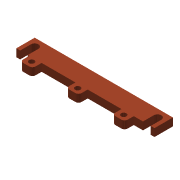
# Autodesk Inventor part: RodHolderV4
Saved by Autodesk Inventor 2013 (Build 170138000, 138)
## iProperties
Created: 2013-04-30
Part Number: RodHolderV4
Material: Copper
Document SubType Name: Modeling
Designer: 120pa
Density: 1 g/cm^3
Author: 120pa
Autodesk Inventor part; units mm, degrees
ref_plane "YZ Plane" through (0, 0, 0) normal (1, 0, 0) x (0, 1, 0)
ref_plane "XZ Plane" through (0, 0, 0) normal (0, 1, 0) x (-1, 0, 0)
ref_plane "XY Plane" through (0, 0, 0) normal (0, 0, 1) x (1, 0, 0)
sketch "Sketch1" plane through (0, 0, 0) normal (0, 1, 0) x (-1, 0, 0)
  line L0 (26.0651, -39.5603) -> (116.0651, -39.5603)
  line L1 (116.0651, -39.5603) -> (116.0651, -27.5603)
  line L2 (116.0651, -27.5603) -> (26.0651, -27.5603)
  line L3 (26.0651, -27.5603) -> (26.0651, -39.5603)
  line L4 (39.5651, -27.5603) -> (47.5651, -27.5603)
  line L5 (47.5651, -27.5603) -> (47.5651, -21.5603)
  line L6 (47.5651, -21.5603) -> (39.5651, -21.5603)
  line L7 (39.5651, -21.5603) -> (39.5651, -27.5603)
  line L8 (69.5651, -27.5603) -> (77.5651, -27.5603)
  line L9 (77.5651, -27.5603) -> (77.5651, -21.5603)
  line L10 (77.5651, -21.5603) -> (69.5651, -21.5603)
  line L11 (69.5651, -21.5603) -> (69.5651, -27.5603)
  line L12 (99.5651, -27.5603) -> (107.5651, -27.5603)
  line L13 (107.5651, -27.5603) -> (107.5651, -21.5603)
  line L14 (107.5651, -21.5603) -> (99.5651, -21.5603)
  line L15 (99.5651, -21.5603) -> (99.5651, -27.5603)
  point P0 (0, 0)
  dimension "d0" = 90
  dimension "d3" = 12
  dimension "d4" = 21.5
  dimension "d5" = 30
  dimension "d6" = 30
  dimension "d7" = 6
  dimension "d8" = 6
  dimension "d9" = 6
  dimension "d10" = 8
  dimension "d11" = 8
  dimension "d12" = 8
  constraints: 32 end point, 8 parallel, 4 horizontal, 4 perpendicular, 3 point on line
  measures "d0" distance of L0.start L0.end
  measures "d3" distance of L0.end L1.end
  measures "d4" distance between parallel lines of L3 L5
  measures "d5" distance between parallel lines of L5 L9
  measures "d6" distance between parallel lines of L9 L13
  measures "d7" distance of L6.end L4.start
  measures "d8" distance of L10.end L8.start
  measures "d9" distance of L14.end L12.start
  measures "d10" distance of L5.end L6.end
  measures "d11" distance of L9.end L10.end
  measures "d12" distance of L13.end L14.end
extrude "Extrusion1" add sketch "Sketch1" along normal blind 5
fillet "Fillet1" radius 2 1 edges at (-99.5651, 2.5, -21.5603)
fillet "Fillet2" radius 2 1 edges at (-107.5651, 2.5, -21.5603)
fillet "Fillet3" radius 2 1 edges at (-77.5651, 2.5, -21.5603)
fillet "Fillet4" radius 2 1 edges at (-69.5651, 2.5, -21.5603)
fillet "Fillet5" radius 2 1 edges at (-47.5651, 2.5, -21.5603)
fillet "Fillet6" radius 2 1 edges at (-39.5651, 2.5, -21.5603)
sketch "Sketch2" plane through (0, 0, 0) normal (0, -1, 0) x (1, 0, 0)
  line L0 (-39.5651, -23.5603) -> (-39.5651, -27.5603) projected
  circle A0 centre (-103.5651, -25.0603) radius 1.75
  circle A1 centre (-73.5651, -25.0603) radius 1.75
  circle A2 centre (-43.5651, -25.0603) radius 1.75
  line L1 (-69.5651, -27.5603) -> (-47.5651, -27.5603) projected
  line L2 (-69.5651, -23.5603) -> (-69.5651, -27.5603) projected
  line L3 (-99.5651, -27.5603) -> (-77.5651, -27.5603) projected
  line L4 (-99.5651, -23.5603) -> (-99.5651, -27.5603) projected
  line L5 (-39.5651, -27.5603) -> (-26.0651, -27.5603) projected
  point P0 (0, 0)
  dimension "d23" = 3.5
  dimension "d29" = 3.5
  dimension "d30" = 3.5
  dimension "d47" = 2.5
  dimension "d48" = 4
  dimension "d49" = 2.5
  dimension "d50" = 4
  dimension "d51" = 2.5
  dimension "d52" = 4
  constraints: 3 centre point
  measures "d23" diameter of A0
  measures "d29" diameter of A1
  measures "d30" diameter of A2
  measures "d47" distance from line of L3 A0.centre
  measures "d48" distance from line of L4 A0.centre
  measures "d49" distance from line of L1 A1.centre
  measures "d50" distance from line of A1.centre L2
  measures "d51" distance from line of L5 A2.centre
  measures "d52" distance from line of L0 A2.centre
extrude "Extrusion2" cut sketch "Sketch2" against normal blind 10
sketch "Sketch4" plane through (0, 5, 0) normal (0, 1, 0) x (1, 0, 0)
  line L0 (-26.0651, 27.5603) -> (-26.0651, 39.5603) projected
  line L1 (-26.0651, 39.5603) -> (-116.0651, 39.5603) projected
  line L2 (-116.0651, 39.5603) -> (-116.0651, 27.5603) projected
  arc A0 (-108.5651, 34.5603) -> (-113.5651, 34.5603) centre (-111.0651, 34.5603) ccw
  arc A1 (-28.5651, 34.5603) -> (-33.5651, 34.5603) centre (-31.0651, 34.5603) ccw
  line L3 (-113.5651, 27.5603) -> (-108.5651, 27.5603)
  line L4 (-108.5651, 27.5603) -> (-108.5651, 34.5603)
  line L5 (-113.5651, 34.5603) -> (-113.5651, 27.5603)
  line L6 (-33.5651, 27.5603) -> (-28.5651, 27.5603)
  line L7 (-28.5651, 27.5603) -> (-28.5651, 34.5603)
  line L8 (-33.5651, 34.5603) -> (-33.5651, 27.5603)
  line L9 (-39.5651, 27.5603) -> (-26.0651, 27.5603) projected
  line L10 (-116.0651, 27.5603) -> (-107.5651, 27.5603) projected
  point P0 (0, 0)
  dimension "d53" = 5
  dimension "d54" = 5
  dimension "d55" = 5
  dimension "d56" = 5
  dimension "d57" = 5
  dimension "d58" = 5
  constraints: 12 end point, 4 point on circle, 4 tangent, 3 point on line, 2 centre point, 1 parallel, 1 perpendicular
  measures "d53" distance from line of L2 A0.centre
  measures "d54" distance from line of L1 A0.centre
  measures "d55" distance between parallel lines of L5 L4
  measures "d56" distance from line of L0 A1.centre
  measures "d57" distance from line of A1.centre L1
  measures "d58" distance between parallel lines of L8 L7
extrude "Extrusion4" cut sketch "Sketch4" against normal blind 10
equation "\"d8\" = d7"
equation "\"d9\" = d7"
body "Solid1"
